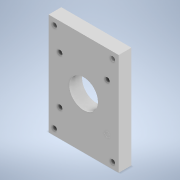
# Autodesk Inventor part: Stepper Mount Y
Saved by Autodesk Inventor 2020 (Build 240168000, 168)
## iProperties
Created: 2020-03-20
Part Number: Stepper Mount Y
Material: Generic
Document SubType Name: Modeling
Designer: DasNick
Density: 1 g/cm^3
Appearance: Default
Author: DasNick
Autodesk Inventor part; units mm, degrees
ref_plane "YZ Plane" through (0, 0, 0) normal (1, 0, 0) x (0, 1, 0)
ref_plane "XZ Plane" through (0, 0, 0) normal (0, 1, 0) x (-1, 0, 0)
ref_plane "XY Plane" through (0, 0, 0) normal (0, 0, 1) x (1, 0, 0)
sketch "Sketch1" plane through (0, 0, 0) normal (0, 0, 1) x (1, 0, 0)
  line L0 (34.925, 6.35) -> (-34.925, 6.35) projected
  line L1 (-34.925, 6.35) -> (-34.925, -6.35) projected
  line L2 (-34.925, -6.35) -> (34.925, -6.35) projected
  line L3 (34.925, -6.35) -> (34.925, 6.35) projected
  circle A0 centre (-29.0032, 0) radius 2.3812 projected
  circle A1 centre (29.0032, 0) radius 2.3812 projected
  line L4 (34.925, -82.55) -> (-34.925, -82.55) projected
  line L5 (-34.925, -82.55) -> (-34.925, -95.25) projected
  line L6 (-34.925, -95.25) -> (34.925, -95.25) projected
  line L7 (34.925, -95.25) -> (34.925, -82.55) projected
  circle A2 centre (-29.0032, -88.9) radius 2.3813 projected
  circle A3 centre (29.0032, -88.9) radius 2.3813 projected
  line L8 (34.925, -6.35) -> (34.925, -82.55)
  line L9 (-34.925, -82.55) -> (-34.925, -6.35)
  point P0 (0, 0)
  constraints: 4 end point, 1 collinear, 1 perpendicular
extrude "Extrusion1" add sketch "Sketch1" along normal blind 12.7
sketch "Sketch2" plane through (0, 0, 12.7) normal (0, 0, 1) x (1, 0, 0)
  circle A0 centre (0, -44.45) radius 14.2875 projected
  point P0 (0, 0)
extrude "Extrusion2" cut sketch "Sketch2" against normal blind 12.7
sketch "Sketch3" plane through (0, 0, 12.7) normal (0, 0, 1) x (1, 0, 0)
  circle A0 centre (23.57, -20.88) radius 2.5 projected
  circle A1 centre (23.57, -68.02) radius 2.5 projected
  circle A2 centre (-23.57, -68.02) radius 2.5 projected
  circle A3 centre (-23.57, -20.88) radius 2.5 projected
  circle A4 centre (23.57, -20.88) radius 2.3812
  circle A5 centre (23.57, -68.02) radius 2.3813
  circle A6 centre (-23.57, -68.02) radius 2.3812
  circle A7 centre (-23.57, -20.88) radius 2.3812
  point P0 (0, 0)
  dimension "d4" = 4.7625
  dimension "d5" = 4.7625
  dimension "d6" = 4.7625
  dimension "d7" = 4.7625
  constraints: 4 centre point, 4 coincident
  measures "d4" diameter of A4
  measures "d5" diameter of A5
  measures "d6" diameter of A6
  measures "d7" diameter of A7
extrude "Extrusion3" cut sketch "Sketch3" against normal blind 25.4 contours A1 | A4 | A6 | A7
body "Solid1"
